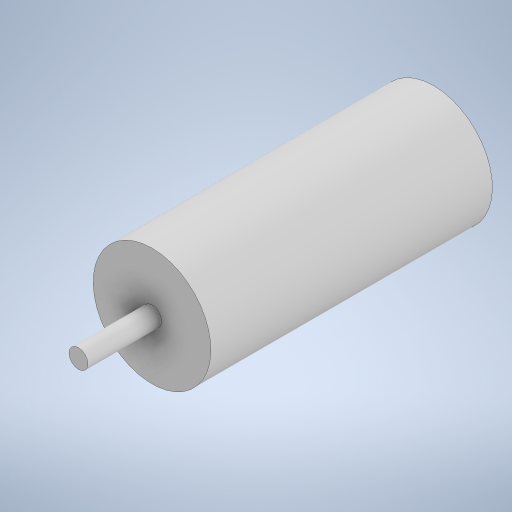
# Autodesk Inventor part: econ gear
Saved by Autodesk Inventor 2023 (Build 270158000, 158)
## iProperties
Created: 2023-01-11
Part Number: econ gear
Material: Generic
Document SubType Name: Modeling
Designer: victo
Density: 1 g/cm^3
Appearance: Default
Author: victo
Autodesk Inventor part; units mm, degrees
ref_plane "YZ Plane" through (0, 0, 0) normal (1, 0, 0) x (0, 1, 0)
ref_plane "XZ Plane" through (0, 0, 0) normal (0, 1, 0) x (-1, 0, 0)
ref_plane "XY Plane" through (0, 0, 0) normal (0, 0, 1) x (1, 0, 0)
sketch "Sketch1" plane through (0, 0, 0) normal (1, 0, 0) x (0, 1, 0)
  line L0 (12.2413, 0.8227) -> (-0.1587, 0.8227)
  line L1 (-0.1587, 0.8227) -> (-0.1587, -58.4773)
  line L2 (-0.1587, -58.4773) -> (12.2413, -58.4773)
  line L3 (12.2413, -58.4773) -> (12.2413, 0.8227)
  line L4 (-0.1587, 0.8227) -> (1.8413, 0.8227)
  line L5 (1.8413, 0.8227) -> (1.8413, 16.3227)
  line L6 (1.8413, 16.3227) -> (-0.1587, 16.3227)
  line L7 (-0.1587, 16.3227) -> (-0.1587, 0.8227)
  line L8 (-0.1587, 23.5633) -> (-0.1587, -69.074)
  point P0 (0, 0)
  dimension "d0" = 59.3
  dimension "d1" = 12.4
  dimension "d2" = 2
  dimension "d3" = 15.5
  constraints: 18 end point, 4 parallel, 2 horizontal, 2 perpendicular, 2 point on line
  measures "d0" distance of L1.end L0.end
  measures "d1" distance between parallel lines of L1 L3
  measures "d2" distance of L6.end L5.end
  measures "d3" distance of L5.end L4.end
revolve "Revolution1" add sketch "Sketch1" angle 360 about axis through (0, -0.1587, 23.5633) along (0, 0, -1)
body "Solid1"
